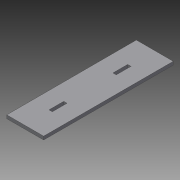
# Autodesk Inventor part: Top
Saved by Autodesk Inventor 2014 (Build 180170000, 170)
## iProperties
Created: 2015-02-09
Part Number: Top
Material: Generic
Document SubType Name: Modeling
Designer: ThatOtherGuy
Density: 1 g/cm^3
Appearance: Default
Author: ThatOtherGuy
Autodesk Inventor part; units mm, degrees
ref_plane "YZ Plane" through (0, 0, 0) normal (1, 0, 0) x (0, 1, 0)
ref_plane "XZ Plane" through (0, 0, 0) normal (0, 1, 0) x (-1, 0, 0)
ref_plane "XY Plane" through (0, 0, 0) normal (0, 0, 1) x (1, 0, 0)
sketch "Sketch1" plane through (0, 0, 0) normal (0, 0, 1) x (1, 0, 0)
  line L0 (0, 0) -> (125, 0)
  line L1 (125, 0) -> (125, 263.462)
  line L2 (125, 263.462) -> (0, 263.462)
  line L3 (0, 263.462) -> (0, 0)
  dimension "d0" = 263.462
  dimension "d1" = 125
  constraints: 8 end point, 2 parallel, 1 horizontal, 1 perpendicular
  measures "d0" distance of L2.end L0.start
  measures "d1" distance of L0.start L0.end
extrude "Extrusion1" add sketch "Sketch1" along normal blind 6.731
sketch "Sketch2" plane through (0, 0, 6.731) normal (0, 0, 1) x (1, 0, 0)
  line L0 (125, 263.462) -> (0, 263.462) projected
  line L1 (0, 263.462) -> (0, 0) projected
  line L2 (59.1345, 211.731) -> (65.8655, 211.731)
  line L3 (65.8655, 211.731) -> (65.8655, 181.731)
  line L4 (65.8655, 181.731) -> (59.1345, 181.731)
  line L5 (59.1345, 181.731) -> (59.1345, 211.731)
  line L6 (59.1345, 81.731) -> (65.8655, 81.731)
  line L7 (65.8655, 81.731) -> (65.8655, 51.731)
  line L8 (65.8655, 51.731) -> (59.1345, 51.731)
  line L9 (59.1345, 51.731) -> (59.1345, 81.731)
  line L10 (62.5, 81.731) -> (62.5, 181.731) construction
  point P0 (62.5, 131.731)
  point P1 (0, 131.731)
  point P2 (62.5, 263.462)
  dimension "d4" = 30
  dimension "d5" = 100
  dimension "d6" = 6.731
  constraints: 18 end point, 5 midpoint, 4 parallel, 2 equal length, 2 horizontal, 2 perpendicular, 1 horizontal alignment, 1 vertical, 1 vertical alignment
  measures "d4" distance of L6.end L7.end
  measures "d5" distance of L10.start L10.end
  measures "d6" distance of L2.start L2.end
extrude "Extrusion2" cut sketch "Sketch2" against normal up to next
sketch "Sketch3" plane through (0, 0, 6.731) normal (0, 0, 1) x (1, 0, 0)
  line L0 (0, 263.462) -> (0, 0) projected
  line L1 (12.5, 19.231) -> (12.5, 49.231) construction
  line L2 (12.5, 49.231) -> (42.5, 49.231) construction
  line L3 (0, 0) -> (125, 0) projected
  point P0 (42.5, 19.231)
  dimension "d9" = 30
  dimension "d10" = 12.5
  dimension "d18" = 19.231
  constraints: 4 end point, 2 horizontal alignment, 2 perpendicular, 2 vertical alignment, 1 parallel
  measures "d9" distance of L1.start L1.end
  measures "d10" distance from line of L0 L1.start
  measures "d18" distance from line of L3 L1.start
hole "Hole1" at (12.5, 49.231, 6.731) at (42.5, 49.231, 6.731) at (42.5, 19.231, 6.731) at (12.5, 19.231, 6.731) direction (0, 0, -1) diameter 16 end through all
equation "\"d2\" = THICKB"
equation "\"d6\" = THICKB"
equation "\"d7\" = THICKB"
equation "\"d18\" = THICKB + d10"
equation "\"THICKA\" = 3.175"
equation "\"THICKB\" = 6.731"
equation "\"THICKC\" = 12.7"
equation "\"THICKPLY\" = 5"
equation "\"MAGDIA\" = 9.5"
equation "\"BALLDIA\" = 12"
body "Solid1"
